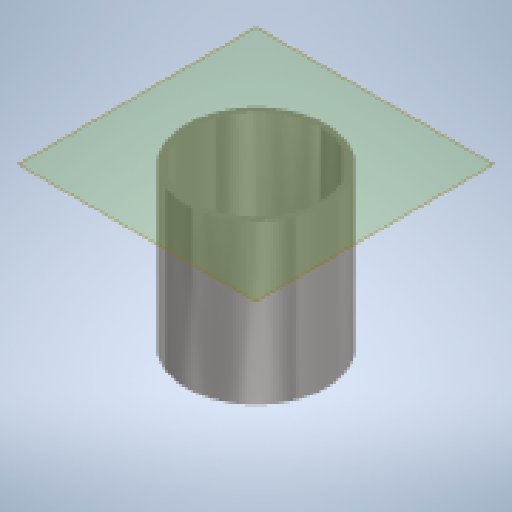
# Autodesk Inventor part: cylinder1
Saved by Autodesk Inventor 2025.2 (Build 292293000, 293)
## iProperties
Created: 2025-03-25
Part Number: cylinder1
Material: Steel, Mild
Document SubType Name: Modeling
Designer: bless
Density: 7.85 g/cm^3
Appearance: Semi-Polished
Author: bless
Autodesk Inventor part; units mm, degrees
ref_plane "YZ Plane" through (0, 0, 0) normal (1, 0, 0) x (0, 1, 0)
ref_plane "XZ Plane" through (0, 0, 0) normal (0, 1, 0) x (-1, 0, 0)
ref_plane "XY Plane" through (0, 0, 0) normal (0, 0, 1) x (1, 0, 0)
ref_plane "Work Plane1" through (-23.3137, -36.6379, -35.1056) normal (0, -1, 0) x (1, 0, 0)
sketch "Sketch1" plane through (-23.3137, -36.6379, -35.1056) normal (0, -1, 0) x (1, 0, 0)
  circle A0 centre (0, 0) radius 97
  circle A1 centre (0, 0) radius 89
  point P0 (23.3137, 35.1056)
  dimension "d0" = 194
  dimension "d1" = 178
  constraints: 2 centre point, 1 coincident
  measures "d0" diameter of A0
  measures "d1" diameter of A1
extrude "Extrusion1" add sketch "Sketch1" along normal blind 220
body "Solid1"
